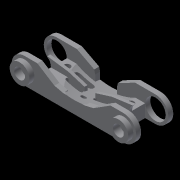
# Autodesk Inventor part: PelvisBaseMount
Saved by Autodesk Inventor 2015 (Build 190159000, 159)
## iProperties
RuleStatus: InUse
Created: 2014-12-04
Part Number: PelvisBaseMount
Material: Generic
Document SubType Name: Modeling
Designer: Val
Density: 1 g/cm^3
Appearance: Default
Mass: 43.7419 g
Surface Area: 190.629 cm^2
Volume: 43.7419 cm^3
BeforeDocSave0: UpdateBoundingBox
CX: 126.00 mm
CY: 42.50 mm
CZ: 26.00 mm
Author: Val
Autodesk Inventor part; units mm, degrees
sketch "Body" plane through (0, 0, 0) normal (0, 0, 1) x (1, 0, 0)
  line L0 (-7.25, -72.7811) -> (-20.75, -72.7811)
  arc A0 (-20.75, -69.2811) -> (-20.75, -72.7811) centre (-20.75, -71.0311) ccw
  line L1 (-8.75, -63.5311) -> (-21.25, -63.5311)
  line L2 (-8.75, -57.0311) -> (-21.25, -57.0311)
  arc A1 (-21.25, -57.0311) -> (-21.25, -63.5311) centre (-21.25, -60.2811) ccw
  arc A2 (-7.25, -72.7811) -> (-7.25, -69.2811) centre (-7.25, -71.0311) ccw
  arc A3 (-8.75, -63.5311) -> (-8.75, -57.0311) centre (-8.75, -60.2811) ccw
  arc A4 (-1, -74.0311) -> (-1, -77.5311) centre (-1, -75.7811) ccw
  circle A5 centre (-32.25, -60.2811) radius 3.25
  line L3 (-18, -66.2811) -> (-18, -69.2811) construction
  line L4 (-18, -48.0311) -> (-18, -53.0311) construction
  line L5 (-40, -66.2811) -> (-5.5, -66.2811)
  line L6 (-5.5, -66.2811) -> (-5.5, -69.2811)
  line L7 (-1, -48.0311) -> (-1, -53.0311)
  line L8 (-63, -80.5311) -> (-40, -80.5311)
  line L9 (-63, -80.5311) -> (-63, -85.5311)
  line L10 (-63, -85.5311) -> (0, -85.5311)
  line L11 (-63, -53.0311) -> (-1, -53.0311)
  line L12 (-63, -48.0311) -> (-63, -53.0311)
  line L13 (-63, -48.0311) -> (-1, -48.0311)
  line L14 (-40, -53.0311) -> (-40, -85.5311)
  line L15 (-60, -53.0311) -> (-60, -80.5311)
  line L16 (0, -85.5311) -> (0, -48.0311)
  line L17 (-1, -48.0311) -> (0, -48.0311)
  line L18 (-1, -74.0311) -> (0, -74.0311)
  line L19 (-1, -77.5311) -> (0, -77.5311)
  line L20 (-20.75, -69.2811) -> (-7.25, -69.2811)
  line L21 (-5.5, -69.2811) -> (-40, -69.2811)
  line L22 (-5.5, -60.2811) -> (-5.5, -71.0311) construction
  line L23 (-32.25, -60.2811) -> (-21.25, -60.2811) construction
  line L24 (0, -93.0311) -> (0, -40.5311) construction
  circle A6 centre (-32.25, -60.2811) radius 5.5 construction
  dimension "d15" = 1.75
  dimension "d16" = 3.25
  dimension "d17" = 20
  dimension "d18" = 3
  dimension "d19" = 63
  dimension "d20" = 5
  dimension "d21" = 5
  dimension "d22" = 3
  dimension "d23" = 13.5
  dimension "d24" = 17
  dimension "d25" = 22
  dimension "d26" = 6.5
  dimension "d29" = 6
  dimension "d30" = 11
  dimension "d31" = 12.5
  dimension "d32" = 1.75
  dimension "d33" = 1
  dimension "d34" = 8
  dimension "d35" = 27.5
  dimension "d67" = 5.5
  dimension "d68" = 11
  constraints: 48 end point, 13 point on circle, 13 point on line, 12 horizontal, 11 tangent, 8 vertical, 7 centre point, 5 collinear, 2 perpendicular, 1 coincident, 1 midpoint
  measures "d15" radius of A0
  measures "d16" radius of A3
  measures "d17" distance between parallel lines of L15 L14
  measures "d18" distance between parallel lines of L12 L15
  measures "d19" distance between parallel lines of L12 L16
  measures "d20" distance between parallel lines of L13 L11
  measures "d21" distance between parallel lines of L10 L8
  measures "d22" distance between parallel lines of L21 L5
  measures "d23" distance of A0.centre A2.centre
  measures "d24" distance between parallel lines of L7 L4
  measures "d25" distance between parallel lines of L14 L3
  measures "d26" diameter of A5
  measures "d29" distance from line of L5 A3.centre
  measures "d30" distance of L23.start L23.end
  measures "d31" distance of L2.start L2.end
  measures "d32" radius of A4
  measures "d33" distance of L18.start L18.end
  measures "d34" distance between parallel lines of L10 L19
  measures "d35" distance of L15.start L15.end
  measures "d67" distance between parallel lines of L24 L22
  measures "d68" diameter of A6
extrude "BodyFeature" add sketch "Body" along normal blind 26 contours A2 L21 L6 L5 L14 L11 L7 L17 L16 L18 A4 L19 L10 A0 L0 | L20 L21 L14 L5 L6 | L14 L8 L15 L11 | L14 L10 L9 L8 | L11 L12 L13 L7
sketch "RoundEnds" plane through (-63, -48.0311, 0) normal (0, 1, 0) x (1, 0, 0)
  arc A0 (13, 0) -> (13, -26) centre (13, -13) ccw
  line L0 (0, 0) -> (0, -26)
  line L1 (13, 0) -> (0, 0)
  line L2 (13, -26) -> (0, -26)
  line L3 (13, 0) -> (0, 0)
  line L4 (0, -26) -> (0, 0)
  line L5 (0, -26) -> (13, -26)
  line L6 (63, 0) -> (0, 0) construction
  line L7 (13, 0) -> (13, -26) construction
  point P0 (0, -13)
  dimension "d131" = 13
  constraints: 16 end point, 3 point on circle, 3 tangent, 2 collinear, 2 perpendicular, 1 centre point, 1 coincident, 1 midpoint, 1 point on line
  measures "d131" radius of A0
extrude "RoundEndsFeature" cut sketch "RoundEnds" against normal through all
sketch "StemMountHole" plane through (0, -48.0311, 26) normal (0, 1, 0) x (1, 0, 0)
  arc A0 (-50, 26) -> (-50, 0) centre (-50, 13) ccw construction
  circle A1 centre (-50, 13) radius 10
  dimension "d40" = 20
  constraints: 1 centre point, 1 coincident
  measures "d40" diameter of A1
hole "StemMountHoleFeature" at (-50, -48.0311, 13) direction (0, -1, 0) diameter 20.5 depth 32.5
sketch "StemMountSideCut" plane through (-60, -80.5311, 4.6934) normal (-1, 0, 0) x (0, 0, 1)
  line L0 (-4.6934, 27.5) -> (21.3066, 27.5)
  line L1 (21.3066, 27.5) -> (21.3066, 0)
  line L2 (21.3066, 0) -> (-4.6934, 0)
  line L3 (-4.6934, 0) -> (-4.6934, 27.5)
  line L4 (0, 27.5) -> (16.6132, 27.5) construction
  line L5 (16.6132, 0) -> (0, 0) construction
  line L6 (10.5566, 27.5) -> (16.6132, 27.5) projected
  line L7 (-4.6934, -5) -> (-4.6934, 32.5) construction
  line L8 (21.3066, -5) -> (21.3066, 32.5) construction
  constraints: 8 end point, 4 collinear, 2 parallel, 1 horizontal, 1 perpendicular
extrude "StemMountSideCutFeature" cut sketch "StemMountSideCut" against normal blind 20.5
sketch "StemBottomMountHole" plane through (0, -85.5311, 0) normal (0, -1, 0) x (1, 0, 0)
  arc A0 (-50, 26) -> (-50, 0) centre (-50, 13) ccw projected
hole "StemBottomMountHoleFeature" at (-50, -85.5311, 13) direction (0, 1, 0) diameter 6.5 end through all counterbore diameter 11 counterbore depth 2
sketch "StemBottomMountCountersinkExtend" plane through (0, -85.5311, 0) normal (0, -1, 0) x (1, 0, 0)
  circle A0 centre (-50, 13) radius 5.5 projected
  circle A1 centre (-50, 13) radius 10
  circle A2 centre (-50, 13) radius 3.25 projected
  dimension "d64" = 20
  constraints: 1 centre point, 1 coincident
  measures "d64" diameter of A1
extrude "StemBottomMountCountersinkExtendFeature" add sketch "StemBottomMountCountersinkExtend" along normal blind 5 contours A1
mirror "AllMirror" about plane through (0, 0, 0) normal (1, 0, 0)
sketch "TopProfile" plane through (-50, -48.0311, 13) normal (0, 1, 0) x (1, 0, 0)
  line L0 (20.5299, -13) -> (38.0299, -3.8993)
  line L1 (38.0299, -3.8993) -> (39, -0.0187)
  line L2 (0, -13) -> (100, -13) construction
  line L3 (39, -0.0187) -> (61, -0.0187)
  line L4 (61, -0.0187) -> (61.9701, -3.8993)
  line L5 (61.9701, -3.8993) -> (79.4701, -13)
  line L6 (20.5299, -13) -> (20.5299, -14)
  line L7 (20.5299, -14) -> (79.4701, -14)
  line L8 (79.4701, -14) -> (79.4701, -13)
  line L9 (0, 13) -> (100, 13) construction
  line L10 (50, 13) -> (50, -13) construction
  point P0 (-13, -13)
  point P1 (113, -13)
  point P2 (-13, 13)
  point P3 (113, 13)
  dimension "d80" = 11
  dimension "d81" = 11
  dimension "d82" = 104.036
  dimension "d83" = 117.476
  dimension "d84" = 1
  dimension "d85" = 104.036
  dimension "d86" = 4
  dimension "d87" = 17.5
  constraints: 18 end point, 2 equal length, 2 horizontal, 2 midpoint, 2 point on line, 1 perpendicular, 1 vertical
  measures "d80" distance from line of L1.end L10
  measures "d81" distance from line of L10 L3.end
  measures "d82" angle of L3 L1
  measures "d83" angle of L0 L6
  measures "d84" distance between parallel lines of L7 L2
  measures "d85" angle of L4 L3
  measures "d86" distance of L0.end L1.end
  measures "d87" horizontal distance of L0.start L0.end
extrude "TopProfileFeature" cut sketch "TopProfile" against normal through all
sketch "MiddleSink" plane through (-11, -48.0311, 13.0187) normal (0, 0, 1) x (1, 0, 0)
  line L0 (-39, -5) -> (-28.5, -5) construction
  line L1 (-28.5, -32.5) -> (-39, -32.5) construction
  line L2 (61, -5) -> (50.5, -5) construction
  line L3 (50.5, -32.5) -> (61, -32.5) construction
  line L4 (-28.5, -5) -> (-28.5, -32.5) construction
  line L5 (50.5, -5) -> (50.5, -32.5) construction
  line L6 (-28.5, -5) -> (50.5, -5)
  line L7 (-28.5, -32.5) -> (50.5, -32.5)
  line L8 (-28.5, -5) -> (-28.5, -32.5)
  line L9 (50.5, -5) -> (50.5, -32.5)
  line L10 (40.4701, 0) -> (40.4701, -37.5) projected
  point P0 (40.4701, -10.5663)
  point P1 (-52, -5)
  point P2 (-52, -32.5)
  point P3 (74, -5)
  point P4 (74, -32.5)
  constraints: 8 end point, 1 horizontal, 1 parallel, 1 perpendicular, 1 vertical
extrude "MiddleSinkFeature" cut sketch "MiddleSink" along normal through all
sketch "BottomProfile" plane through (-50, -80.5311, 13) normal (0, 1, 0) x (1, 0, 0)
  line L0 (13, -17) -> (41.8345, -17)
  line L1 (30.2369, -2.0701) -> (39, -0.0187)
  line L2 (39, -0.0187) -> (41.8345, -17)
  arc A0 (0, 13) -> (0, -13) centre (0, 0) ccw construction
  circle A1 centre (0, 0) radius 13 construction
  line L3 (39, -0.0187) -> (10.5, -0.0187) construction
  line L4 (13, -0.0187) -> (13, -13) construction
  line L5 (20.5299, -13) -> (0, -13) construction
  line L6 (13, -13) -> (30.2369, -2.0701)
  line L7 (13, -13) -> (13, -17)
  line L8 (20.5299, -13) -> (38.0299, -3.8993) construction
  line L9 (61, -0.0187) -> (39, -0.0187) construction
  line L10 (50, -0.0187) -> (50, 13) construction
  line L11 (0, 13) -> (100, 13) construction
  line L12 (87, -17) -> (58.1655, -17)
  line L13 (69.7631, -2.0701) -> (61, -0.0187)
  line L14 (61, -0.0187) -> (58.1655, -17)
  line L15 (87, -13) -> (69.7631, -2.0701)
  line L16 (87, -13) -> (87, -17)
  point P0 (-13, -13)
  point P1 (-13, 13)
  point P2 (113, 13)
  dimension "d94" = 4
  dimension "d97" = 9
  dimension "d98" = 72
  dimension "d99" = 20.4101
  constraints: 24 end point, 4 symmetric about line, 2 midpoint, 2 perpendicular, 2 point on circle, 2 point on line, 1 centre point, 1 coincident, 1 collinear, 1 horizontal
  measures "d94" distance between parallel lines of L0 L5
  measures "d97" distance of L1.start L1.end
  measures "d98" angle of L2 L8
  measures "d99" distance of L4.end L1.start
extrude "BottomProfileFeature" cut sketch "BottomProfile" against normal through all
ref_plane "MiddleRidgePlane" through (-5.5, -69.2811, 0) normal (0, 1, 0) x (1, 0, 0)
sketch "MiddleRidge" plane through (-5.5, -69.2811, 0) normal (0, 1, 0) x (1, 0, 0)
  line L0 (-23.9701, -26) -> (-6.4701, -16.8993) construction
  line L1 (34.9701, -26) -> (-23.9701, -26) construction
  line L2 (0, -13.0187) -> (-16.75, -18.1397)
  line L3 (16.5, -13.0187) -> (-5.5, -13.0187) construction
  circle A0 centre (-44.5, -13) radius 10.5 construction
  circle A1 centre (-44.5, -13) radius 10 construction
  line L4 (0, -13.0187) -> (-34, -13.0187)
  line L5 (-16.75, -18.1397) -> (-37.7213, -21.0187)
  arc A2 (-37.7213, -21.0187) -> (-34, -13.0187) centre (-44.5, -13) ccw
  line L6 (-1.75, -13.0187) -> (0, -13.0187) projected
  line L7 (6.5, -13.0187) -> (4.5, -13.0187) construction
  line L8 (4.5, -13.0187) -> (6.5, -13.0187) construction
  line L9 (5.5, -13.0187) -> (5.5, -8.0187) construction
  line L10 (11, -13.0187) -> (27.75, -18.1397)
  line L11 (11, -13.0187) -> (45, -13.0187)
  line L12 (27.75, -18.1397) -> (48.7213, -21.0187)
  arc A3 (45, -13.0187) -> (48.7213, -21.0187) centre (55.5, -13) ccw
  line L13 (-17, -13.0187) -> (-15.25, -13.0187) projected
  line L14 (-15.25, 0) -> (-15.25, -13.0187) construction
  point P0 (-44.5, -26)
  dimension "d105" = 0.5
  dimension "d107" = 17
  dimension "d110" = 5
  dimension "d111" = 1.5
  dimension "d112" = 8
  constraints: 14 end point, 6 point on circle, 5 symmetric about line, 3 centre point, 2 concentric, 1 horizontal, 1 midpoint, 1 vertical, 1 other
  measures "d105" radial gap between concentric circles of A1 A0
  measures "d107" angle of L4 L2
  measures "d110" distance of L9.start L9.end
  measures "d111" distance from line of L2.end L14
  measures "d112" vertical distance of L4.end L5.end
extrude "MiddleRidgeFeature" add sketch "MiddleRidge" along normal up to surface (3 mm away) separate body
ref_plane "TopRidgesSplitPlane" through (-39.5, -53.0311, 13.0187) normal (0, 0, 1) x (1, 0, 0)
split body "TopRidgesSplitFeature" result two bodies by plane through (-39.5, -53.0311, 13.0187) normal (0, 0, 1) bodies 1 first body at (-32.3525, -85.0311, 18.8262) (32.3525, -85.0311, 18.8262) (27.0634, -48.5311, 18.6393) (-27.0634, -48.5311, 18.6393)
ref_plane "MiddlePlane" through (0, -80.5311, 0) normal (1, 0, 0) x (0, 0, -1)
sketch "MiddleIndent" plane through (0, -80.5311, 0) normal (1, 0, 0) x (0, 0, -1)
  arc A0 (-87.3745, -188.4762) -> (-24.2483, -39.7825) centre (-7034.1024, 2848.4227) ccw
  arc A1 (-24.2483, -39.7825) -> (-57.3731, 236.5622) centre (-287.7578, 68.7888) ccw
  line L0 (-87.3745, -188.4762) -> (-57.3731, 236.5622)
  dimension "d125" = 285
  dimension "d126" = 7581.5423
  dimension "d127" = 52.5
  dimension "d128" = 218
  constraints: 4 point on circle, 2 centre point, 2 end point, 1 tangent
  measures "d125" radius of A1
  measures "d126" radius of A0
  measures "d127" distance from line of A0.end L0
  measures "d128" distance from line of A1.centre L0
revolve "MiddleIndentFeature" cut sketch "MiddleIndent" angle 360 about axis through (0, -269.0073, 87.3745) along (0, 0.9975181, -0.0704098) bodies 4
combine bodies "CombineRidgesFeature" operation type add bodies to combine 3 2
sketch "ExtendRidges" plane through (-11, -85.5311, 13.0187) normal (0, 0, -1) x (-1, 0, 0)
  line L0 (29, 0) -> (29, 5)
  line L1 (35.7501, 5) -> (28.5, 5) construction
  line L2 (29, 0) -> (29, -5) construction
  line L3 (29, 5) -> (0, 5)
  line L4 (0, 5) -> (0, 0)
  line L5 (0, 0) -> (29, 0)
  line L6 (-22, 5) -> (-22, 0)
  line L7 (-22, 0) -> (-51, 0)
  line L8 (-51, 0) -> (-51, 5)
  line L9 (-22, 5) -> (-51, 5)
  line L10 (-50.5, 5) -> (-22, 5) projected
  line L11 (28.5, 19.25) -> (-5.5, 19.25) projected
  line L12 (-5.5, 16.25) -> (-5.5, 19.25) projected
  line L13 (-5.5, 16.25) -> (28.5, 16.25) projected
  line L14 (28.5, 16.25) -> (28.5, 19.25) projected
  line L15 (-16.5, 19.25) -> (-50.5, 19.25) projected
  line L16 (-50.5, 16.25) -> (-50.5, 19.25) projected
  line L17 (-16.5, 16.25) -> (-50.5, 16.25) projected
  line L18 (-16.5, 16.25) -> (-16.5, 19.25) projected
  line L19 (0, 37.5) -> (0, 32.5) projected
  line L20 (28.5, 32.5) -> (0, 32.5) projected
  line L21 (28.5, 32.5) -> (28.75, 32.5) projected
  line L22 (28.75, 32.5) -> (28.75, 37.5) projected
  line L23 (28.75, 37.5) -> (0, 37.5) projected
  line L24 (-22, 32.5) -> (-50.5, 32.5) projected
  line L25 (-22, 37.5) -> (-22, 32.5) projected
  line L26 (-22, 37.5) -> (-50.75, 37.5) projected
  line L27 (-50.75, 37.5) -> (-50.75, 32.5) projected
  line L28 (-50.75, 32.5) -> (-50.5, 32.5) projected
  constraints: 16 end point, 3 perpendicular, 2 collinear, 2 vertical, 1 horizontal, 1 point on line
extrude "ExtendRidgesFeature" add sketch "ExtendRidges" along normal blind 10 bodies 3
combine bodies "CombineRidgesAndBodyFeature" operation type add bodies to combine 3 4
equation "\"d81\" = d80"
equation "\"d85\" = d82"
body "Solid6"
